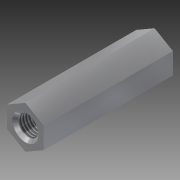
# Autodesk Inventor part: CNC- Hexagonal Bit
Saved by Autodesk Inventor 2015 (Build 190159000, 159)
## iProperties
Created: 2015-03-21
Part Number: CNC- Hexagonal Bit
Material: Generic
Document SubType Name: Modeling
Designer: Bangladesh
Density: 1 g/cm^3
Appearance: Default
Author: Bangladesh
Autodesk Inventor part; units mm, degrees
ref_plane "YZ Plane" through (0, 0, 0) normal (1, 0, 0) x (0, 1, 0)
ref_plane "XZ Plane" through (0, 0, 0) normal (0, 1, 0) x (-1, 0, 0)
ref_plane "XY Plane" through (0, 0, 0) normal (0, 0, 1) x (1, 0, 0)
sketch "Sketch1" plane through (0, 0, 0) normal (0, 0, 1) x (1, 0, 0)
  circle A0 centre (0, 0) radius 7.255
  line L0 (0, -7.255) -> (-6.283, -3.6275)
  line L1 (-6.283, -3.6275) -> (-6.283, 3.6275)
  line L2 (-6.283, 3.6275) -> (0, 7.255)
  line L3 (0, 7.255) -> (6.283, 3.6275)
  line L4 (6.283, 3.6275) -> (6.283, -3.6275)
  line L5 (6.283, -3.6275) -> (0, -7.255)
  dimension "d0" = 14.51
  constraints: 12 end point, 2 coincident, 1 vertical alignment, 15 other
extrude "Extrusion1" add sketch "Sketch1" along normal mid plane 44.28 contours L4 L5 L0 L1 L2 L3
sketch "Sketch2" plane through (0, 0, 22.14) normal (0, 0, 1) x (1, 0, 0)
  circle A0 centre (0, 0) radius 4.3621
  constraints: 1 centre point, 1 coincident
hole "Hole1" at (0, 0, 22.14) direction (0, 0, -1) diameter 6.9088 end through all
chamfer "Chamfer1" distance 1 angle 45 1 edges at (0, 3.4544, 22.14)
chamfer "Chamfer2" distance 1 angle 45 1 edges at (0, 3.4544, -22.14)
body "Solid1"
